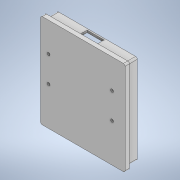
# Autodesk Inventor part: Cubierta parte 1
Saved by Autodesk Inventor 2021 (Build 250183000, 183)
## iProperties
Created: 2021-08-03
Part Number: Cubierta parte 1
Material: Generic
Document SubType Name: Modeling
Designer: Admin
Density: 1 g/cm^3
Appearance: Default
Author: Admin
Autodesk Inventor part; units mm, degrees
ref_plane "YZ Plane" through (0, 0, 0) normal (1, 0, 0) x (0, 1, 0)
ref_plane "XZ Plane" through (0, 0, 0) normal (0, 1, 0) x (-1, 0, 0)
ref_plane "XY Plane" through (0, 0, 0) normal (0, 0, 1) x (1, 0, 0)
sketch "Sketch1" plane through (0, 0, 0) normal (0, 0, 1) x (1, 0, 0)
  line L0 (-44.577, -50) -> (44.577, -50) projected
  line L1 (44.577, -50) -> (44.577, 50) projected
  line L2 (44.577, 50) -> (-44.577, 50) projected
  line L3 (-44.577, 50) -> (-44.577, -50) projected
  line L4 (49.577, 55) -> (49.577, -55)
  line L5 (49.577, -55) -> (-49.577, -55)
  line L6 (-49.577, -55) -> (-49.577, 55)
  line L7 (-49.577, 55) -> (49.577, 55)
  circle A0 centre (34.337, -9.9) radius 1.7 projected
  circle A1 centre (34.337, 20.6) radius 1.7 projected
  circle A2 centre (-40.163, -9.9) radius 1.7 projected
  circle A3 centre (-40.163, 20.6) radius 1.7 projected
  point P0 (0, 0)
  dimension "d0" = 5
  constraints: 8 end point, 3 other
  measures "d0" distance between parallel lines of L4 L1
extrude "Extrusion1" add sketch "Sketch1" along normal blind 5 contours L3 L2 L1 L0 | L4 L5 L6 L7
sketch "Sketch2" plane through (0, 0, 0) normal (0, 0, -1) x (-1, 0, 0)
  line L0 (44.577, -50) -> (-44.577, -50) projected
  line L1 (44.577, 50) -> (44.577, -50) projected
  line L2 (-44.577, 50) -> (44.577, 50) projected
  line L3 (-44.577, -50) -> (-44.577, 50) projected
  line L4 (49.577, 55) -> (49.577, -55) projected
  line L5 (-49.577, 55) -> (49.577, 55) projected
  line L6 (-49.577, -55) -> (-49.577, 55) projected
  line L7 (49.577, -55) -> (-49.577, -55) projected
  circle A0 centre (-34.337, -9.9) radius 1.7 projected
  circle A1 centre (-34.337, 20.6) radius 1.7 projected
  circle A2 centre (40.163, -9.9) radius 1.7 projected
  circle A3 centre (40.163, 20.6) radius 1.7 projected
  line L8 (44.577, 50) -> (44.577, -50)
  line L9 (44.577, -50) -> (-44.577, -50)
  line L10 (-44.577, -50) -> (-44.577, 50)
  line L11 (-44.577, 50) -> (44.577, 50)
  line L12 (47.077, 52.5) -> (47.077, -52.5)
  line L13 (47.077, -52.5) -> (-47.077, -52.5)
  line L14 (-47.077, -52.5) -> (-47.077, 52.5)
  line L15 (-47.077, 52.5) -> (47.077, 52.5)
  point P0 (0, 0)
  dimension "d3" = 0
  dimension "d4" = 2.5
  constraints: 16 end point, 6 other
  measures "d3" distance between parallel lines of L11 L2
  measures "d4" distance between parallel lines of L5 L15
extrude "Extrusion2" add sketch "Sketch2" along normal blind 11.75 contours L12 L13 L14 L15
fillet "Fillet1" radius 2 7 edges at (47.077, -52.5, -5.875) (49.577, -55, 2.5) (-49.577, -55, 2.5) (-49.577, 55, 2.5) (-47.077, 52.5, -5.875) (47.077, 52.5, -5.875) (49.577, 55, 2.5)
sketch "Sketch3" plane through (-47.077, -52.5, -11.75) normal (0, -1, 0) x (1, 0, 0)
  line L0 (39.1897, 5.1489) -> (39.1897, 11.75) projected
  line L1 (55.1104, 5.1489) -> (39.1897, 5.1489) projected
  line L2 (55.1104, 11.75) -> (55.1104, 5.1489) projected
  line L3 (0, 11.75) -> (92.154, 11.75) projected
  point P0 (47.077, 11.75)
extrude "Extrusion3" cut sketch "Sketch3" against normal blind 11.75
sketch "Sketch4" plane through (-45.077, 52.5, 0) normal (0, 1, 0) x (1, 0, 0)
  line L0 (35.077, 10) -> (55.077, 10) projected
  line L1 (35.077, 0) -> (35.077, 10) projected
  line L2 (55.077, 10) -> (55.077, 0) projected
  line L3 (90.154, 0) -> (0, 0) projected
  point P0 (45.077, 0)
extrude "Extrusion4" cut sketch "Sketch4" against normal blind 11.75
body "Solid1"
